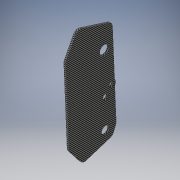
# Autodesk Inventor part: Module Plate 1
Saved by Autodesk Inventor 2019.4 (Build 234330000, 330)
## iProperties
Created: 2019-10-19
Part Number: Module Plate 1
Material: CFRP
Document SubType Name: Modeling
Designer: admin
Density: 1.43 g/cm^3
Appearance: Carbon Fiber
d27: 7.000 mm
Height: 80.000 mm
Author: admin
Autodesk Inventor part; units mm, degrees
ref_plane "YZ Plane" through (0, 0, 0) normal (1, 0, 0) x (0, 1, 0)
ref_plane "XZ Plane" through (0, 0, 0) normal (0, 1, 0) x (-1, 0, 0)
ref_plane "XY Plane" through (0, 0, 0) normal (0, 0, 1) x (1, 0, 0)
sketch "Sketch1" plane through (0, 0, 0) normal (1, 0, 0) x (0, 1, 0)
  circle A0 centre (0, 0) radius 62.5 construction
  circle A1 centre (-146.0656, -2.5) radius 50 construction
  line L0 (-146.0656, -2.5) -> (0, 0) construction
  line L1 (-172.7208, -52.5) -> (-113.4241, -52.5) construction
  line L2 (-16.0459, -62.5) -> (40.9165, -62.5) construction
  line L3 (-162.86, -17.263) -> (-144.3319, -24.7934)
  line L4 (-144.3319, -24.7934) -> (-74.6779, -21.7515)
  line L5 (41.9313, -16.659) -> (64.9582, 56.3758)
  line L6 (64.9582, 56.3758) -> (17.9251, 80.8591)
  line L7 (17.9251, 80.8591) -> (-145.8225, 73.708)
  line L8 (-145.8225, 73.708) -> (-182.9035, 44.86)
  line L9 (-182.9035, 44.86) -> (-162.86, -17.263)
  circle A2 centre (0, 0) radius 9.8
  circle A3 centre (-146.0656, -2.5) radius 8.3
  line L10 (-153.5959, -21.0282) -> (-146.0656, -2.5) construction
  arc A4 (-74.6779, -21.7515) -> (-63.375, -21.2579) centre (-69.3319, -14.5113) ccw
  arc A5 (-63.375, -21.2579) -> (-74.6779, -21.7515) centre (-69.3319, -14.5113) ccw construction
  line L11 (-99.9551, -22.8554) -> (-99.3168, -22.8275) construction
  line L12 (-99.3168, -22.8275) -> (-63.375, -21.2579) construction
  line L13 (-74.6779, -21.7515) -> (-99.9551, -22.8554) construction
  line L14 (-63.375, -21.2579) -> (41.9313, -16.659)
  circle A6 centre (-69.3319, -14.5113) radius 4.3
  line L15 (0, 0) -> (-212.6616, 0) construction
  circle A7 centre (-86.0656, -2.2297) radius 5.3
  dimension "d0" = 125
  dimension "d1" = 100
  dimension "d2" = 146.087
  dimension "d3" = 10
  dimension "d4" = 20
  dimension "d5" = 19.6
  dimension "d6" = 16.6
  dimension "d7" = 23.099
  dimension "d8" = 20
  dimension "d9" = 130
  dimension "d10" = 110
  dimension "d12" = 155.381
  dimension "d13" = 80
  dimension "d14" = 100
  dimension "d15" = 150
  dimension "Height" = 80
  dimension "d17" = 45
  dimension "d18" = 60
  dimension "d19" = 18
  dimension "d26" = 8.6
  dimension "d27" = 7
  dimension "d28" = 75
  dimension "d30" = 10.6
  dimension "d31" = 20
  dimension "d32" = 60
  constraints: 32 end point, 8 centre point, 5 parallel, 4 coincident, 4 point on circle, 3 horizontal, 2 point on line, 2 tangent, 1 midpoint, 1 perpendicular
  measures "d0" diameter of A0
  measures "d1" diameter of A1
  measures "d2" distance of L0.start L0.end
  measures "d3" distance between parallel lines of L2 L1
  measures "d4" distance from line of L0.start L3
  measures "d5" diameter of A2
  measures "d6" diameter of A3
  measures "d7" angle of L0 L3
  measures "d8" distance of L3.start L3.end
  measures "d9" angle of L3 L9
  measures "d10" angle of L9 L8
  measures "d12" angle of L4 L3
  measures "d13" distance from line of L15.start L7
  measures "d14" angle of L5 L6
  measures "d15" angle of L7 L6
  measures "Height" distance from line of point (0, 0) L6
  measures "d17" distance from line of L15.start L5
  measures "d18" distance from line of L10.end L8
  measures "d19" diameter of A4
  measures "d26" diameter of A6
  measures "d27" distance from line of L4 A6.centre
  measures "d28" horizontal distance of L3.end A6.centre
  measures "d30" diameter of A7
  measures "d31" distance from line of L4 A7.centre
  measures "d32" horizontal distance of L0.start A7.centre
extrude "Extrusion1" add sketch "Sketch1" along normal blind 4
fillet "Fillet1" radius 2 2 edges at (2, -74.6779, -21.7515) (2, -63.375, -21.2579)
fillet "Fillet2" radius 10 7 edges at (2, -182.9035, 44.86) (2, -145.8225, 73.708) (2, -162.86, -17.263) (2, 17.9251, 80.8591) (2, 64.9582, 56.3758) (2, 41.9313, -16.659) (2, -144.3319, -24.7934)
body "Solid1"
